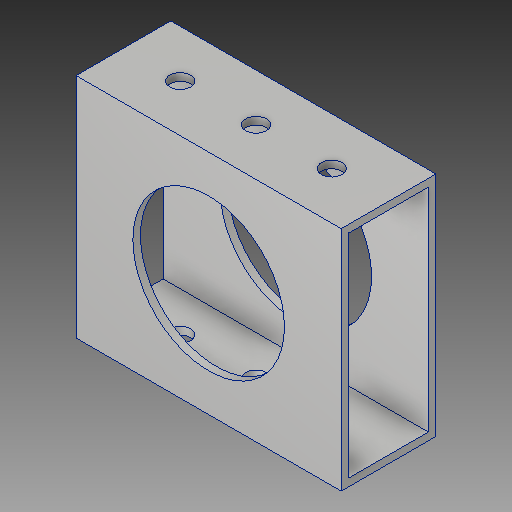
# Autodesk Inventor part: Bumper Support
Saved by Autodesk Inventor 2019.4 (Build 234330000, 330)
## iProperties
Created: 2019-12-12
Part Number: Bumper Support
Material: Aluminum 6061
Document SubType Name: Modeling
Designer: admin
Density: 2.7 g/cm^3
Appearance: Aluminum - Flat
Author: admin
Autodesk Inventor part; units mm, degrees
ref_plane "YZ Plane" through (0, 0, 0) normal (1, 0, 0) x (0, 1, 0)
ref_plane "XZ Plane" through (0, 0, 0) normal (0, 1, 0) x (-1, 0, 0)
ref_plane "XY Plane" through (0, 0, 0) normal (0, 0, 1) x (1, 0, 0)
sketch "Sketch1" plane through (0, 0, 0) normal (1, 0, 0) x (0, 1, 0)
  line L0 (-30, 12.5) -> (30, 12.5)
  line L1 (30, 12.5) -> (30, -12.5)
  line L2 (30, -12.5) -> (-30, -12.5)
  line L3 (-30, -12.5) -> (-30, 12.5)
  line L4 (-30, 12.5) -> (30, -12.5) construction
  line L5 (30, 12.5) -> (-30, -12.5) construction
  line L6 (28, -10.5) -> (28, 10.5)
  line L7 (28, 10.5) -> (-28, 10.5)
  line L8 (-28, 10.5) -> (-28, -10.5)
  line L9 (-28, -10.5) -> (28, -10.5)
  point P0 (0, 0)
  dimension "d0" = 60
  dimension "d1" = 25
  dimension "d2" = 2
  constraints: 20 end point, 4 parallel, 2 midpoint, 2 perpendicular, 1 horizontal, 3 other
  measures "d0" distance of L1.end L2.end
  measures "d1" distance of L0.end L1.end
  measures "d2" distance between parallel lines of L1 L6
extrude "Extrusion1" add sketch "Sketch1" along normal blind 70
sketch "Sketch2" plane through (0, 30, 12.5) normal (0, 1, 0) x (1, 0, 0)
  circle A0 centre (15, 12.5) radius 2.75
  circle A1 centre (35, 12.5) radius 2.75
  circle A2 centre (55, 12.5) radius 2.75
  line L0 (0, 0) -> (0, 25) projected
  line L1 (15, 12.5) -> (55, 12.5) construction
  point P0 (0, 12.5)
  point P1 (0, 12.5)
  dimension "d5" = 5.5
  dimension "d6" = 5.5
  dimension "d7" = 5.5
  dimension "d8" = 20
  dimension "d9" = 20
  dimension "d10" = 15
  dimension "d11" = 40
  constraints: 3 centre point, 2 end point, 1 horizontal, 1 midpoint, 1 point on line
  measures "d5" diameter of A0
  measures "d6" diameter of A1
  measures "d7" diameter of A2
  measures "d8" distance of A1.centre L1.start
  measures "d9" distance of L1.end A1.centre
  measures "d10" distance from line of L0 L1.start
  measures "d11" distance of L1.start L1.end
extrude "Extrusion2" cut sketch "Sketch2" against normal through all
sketch "Sketch3" plane through (0, -30, 12.5) normal (0, 0, 1) x (1, 0, 0)
  circle A0 centre (35, 30) radius 20
  line L0 (70, 60) -> (70, 0) projected
  line L1 (0, 0) -> (70, 0) projected
  point P0 (0, 30)
  dimension "d14" = 40
  dimension "d15" = 35
  dimension "d16" = 30
  constraints: 1 centre point
  measures "d14" diameter of A0
  measures "d15" distance from line of L0 A0.centre
  measures "d16" distance from line of L1 A0.centre
extrude "Extrusion3" cut sketch "Sketch3" against normal blind 30
body "Solid1"
